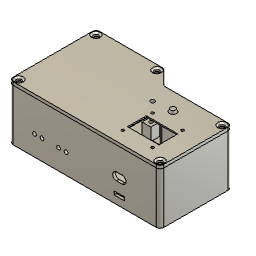
Blender_Box (Autodesk Fusion 360 design; units mm, degrees)
Autodesk Fusion 360 part; units mm, degrees
note: some values were not read from the file. Set by a fixed rule: which face or edge a step refers to.
sketch "Sketch1" plane through (0, 0, 0) normal (0, 1, 0) x (1, 0, 0)
  line L0 (0, 0) -> (120, 0)
  line L1 (0, 0) -> (0, 69)
  line L2 (0, 69) -> (54, 69)
  line L3 (54, 69) -> (66, 57)
  line L4 (66, 57) -> (120, 57)
  line L5 (120, 57) -> (120, 0)
  line L6 (54, 69) -> (54, 0) construction
  line L7 (66, 57) -> (66, 0) construction
  dimension "d1" = 120
  dimension "d2" = 69
  dimension "d3" = 54
  dimension "d5" = 57
  dimension "d28" = 54
  constraint coincident L0.start L1.start
  constraint horizontal L0
  constraint perpendicular L0 L1
  constraint perpendicular L1 L2
  constraint perpendicular L1 L4
  constraint perpendicular L0 L5
  constraint perpendicular L0 L6
  constraint coincident L0 L7.end
  constraint perpendicular L0 L7
  measures "d1" distance of L0.start L0.end
  measures "d2" distance of L0 L2
  measures "d3" distance of L1 L6
  measures "d5" distance of L0 L4
  measures "d28" distance of L5 L7
extrude "Extrude1" add sketch "Sketch1" along normal blind 41 makes body 1
shell "Shell1" thickness 2 removed faces 1 at (62, 41, -19) on bodies 1
sketch "Sketch2" plane through (0, 41, 0) normal (0, 1, 0) x (-1, 0, 0)
  line L0 (-2, -2) -> (-2, -67)
  line L1 (-2, -67) -> (-53.1716, -67)
  line L2 (-53.1716, -67) -> (-65.1716, -55)
  line L3 (-65.1716, -55) -> (-118, -55)
  line L4 (-118, -55) -> (-118, -2)
  line L5 (-118, -2) -> (-2, -2)
  line L6 (0, 0) -> (-120, 0)
  line L7 (-120, 0) -> (-120, -57)
  line L8 (-120, -57) -> (-66, -57)
  line L9 (-66, -57) -> (-54, -69)
  line L10 (-54, -69) -> (0, -69)
  line L11 (0, -69) -> (0, 0)
  circle A0 centre (-3.85, -3.85) radius 1.85
  circle A1 centre (-3.85, -65.15) radius 1.85
  circle A2 centre (-52.4053, -65.15) radius 1.85
  circle A3 centre (-116.15, -53.15) radius 1.85
  circle A4 centre (-116.15, -3.85) radius 1.85
  circle A5 centre (-3.85, -65.15) radius 3.85
  circle A6 centre (-52.4053, -65.15) radius 3.85
  circle A7 centre (-3.85, -3.85) radius 3.85
  circle A8 centre (-116.15, -53.15) radius 3.85
  circle A9 centre (-116.15, -3.85) radius 3.85
  dimension "d10" = 3.7
  constraint tangent L4 A4
  constraint tangent L5 A4
  constraint tangent L3 A3
  constraint tangent L4 A3
  constraint tangent L1 A2
  constraint tangent L2 A2
  constraint tangent L1 A1
  constraint tangent L0 A1
  constraint tangent L0 A0
  constraint tangent L5 A0
  constraint equal A0 A1
  constraint equal A0 A2
  constraint equal A2 A3
  constraint equal A3 A4
  constraint concentric A1 A5
  constraint concentric A2 A6
  constraint concentric A0 A7
  constraint concentric A3 A8
  constraint concentric A4 A9
  constraint tangent L7 A9
  constraint tangent L8 A8
  constraint tangent L9 A6
  constraint tangent L10 A5
  constraint tangent L11 A7
  measures "d10" diameter of A2
extrude "Extrude2" add sketch "Sketch2" against normal up to surface (39 mm away) contours L0 L5 A0 | L0 L5 A0 A7 | L0 L1 A1 A5 | L4 L5 A4 A9 | L0 L1 A1 | L4 L5 A4 | L1 L2 A2 A6 | L1 L2 A2 | L3 L4 A3 A8 | L3 L4 A3 bodies 1
fillet "Fillet1" radius 3 17 edges at (7.2264, 21.5, -67) (2, 21.5, -61.7736) (49.0289, 21.5, -67) (56.1009, 21.5, -64.0707) (65.1716, 21.5, -55) (112.7736, 21.5, -55) (118, 21.5, -49.7736) (0, 20.5, 0) (0, 20.5, -69) (54, 20.5, -69) (66, 20.5, -57) (120, 20.5, -57) (112.7736, 21.5, -2) (118, 21.5, -7.2264) (120, 20.5, 0) (7.2264, 21.5, -2) (2, 21.5, -7.2264) on bodies 1
sketch "Sketch4" plane through (0, 41, 0) normal (0, 1, 0) x (-1, 0, 0)
  arc A0 (-117, 0) -> (-120, -3) centre (-117, -3) ccw
  line L0 (-120, -3) -> (-120, -54)
  arc A1 (-120, -54) -> (-117, -57) centre (-117, -54) ccw
  line L1 (-117, -57) -> (-67.2426, -57)
  arc A2 (-65.1213, -57.8787) -> (-67.2426, -57) centre (-67.2426, -60) ccw
  line L2 (-65.1213, -57.8787) -> (-54.8787, -68.1213)
  arc A3 (-54.8787, -68.1213) -> (-52.7574, -69) centre (-52.7574, -66) ccw
  line L3 (-52.7574, -69) -> (-3, -69)
  arc A4 (-3, -69) -> (0, -66) centre (-3, -66) ccw
  line L4 (0, -66) -> (0, -3)
  arc A5 (0, -3) -> (-3, 0) centre (-3, -3) ccw
  line L5 (-3, 0) -> (-117, 0)
  circle A6 centre (-116.15, -3.85) radius 1.85
  circle A7 centre (-3.85, -65.15) radius 1.85
  circle A8 centre (-3.85, -3.85) radius 1.85
  circle A9 centre (-52.4053, -65.15) radius 1.85
  circle A10 centre (-116.15, -53.15) radius 1.85
  arc A11 (-64.2929, -55.8787) -> (-66.4142, -55) centre (-66.4142, -58) ccw
  line L6 (-66.4142, -55) -> (-109.3972, -55)
  arc A12 (-112.3546, -52.5036) -> (-109.3972, -55) centre (-109.3972, -52) ccw
  arc A13 (-112.3546, -52.5036) -> (-115.5036, -49.3546) centre (-116.15, -53.15) ccw
  arc A14 (-118, -46.3972) -> (-115.5036, -49.3546) centre (-115, -46.3972) ccw
  line L7 (-118, -46.3972) -> (-118, -10.6028)
  arc A15 (-115.5036, -7.6454) -> (-118, -10.6028) centre (-115, -10.6028) ccw
  arc A16 (-115.5036, -7.6454) -> (-112.3546, -4.4964) centre (-116.15, -3.85) ccw
  arc A17 (-109.3972, -2) -> (-112.3546, -4.4964) centre (-109.3972, -5) ccw
  line L8 (-109.3972, -2) -> (-10.6028, -2)
  arc A18 (-7.6454, -4.4964) -> (-4.4964, -7.6454) centre (-3.85, -3.85) ccw
  line L9 (-2, -10.6028) -> (-2, -58.3972)
  arc A19 (-4.4964, -61.3546) -> (-2, -58.3972) centre (-5, -58.3972) ccw
  arc A20 (-4.4964, -61.3546) -> (-7.6454, -64.5036) centre (-3.85, -65.15) ccw
  arc A21 (-10.6028, -67) -> (-7.6454, -64.5036) centre (-10.6028, -64) ccw
  line L10 (-10.6028, -67) -> (-45.6525, -67)
  arc A22 (-48.6099, -64.5036) -> (-45.6525, -67) centre (-45.6525, -64) ccw
  arc A23 (-48.6099, -64.5036) -> (-54.632, -62.0092) centre (-52.4053, -65.15) ccw
  arc A24 (-58.4884, -61.6832) -> (-54.632, -62.0092) centre (-56.367, -59.5619) ccw
  line L11 (-58.4884, -61.6832) -> (-64.2929, -55.8787)
  arc A25 (-7.6454, -4.4964) -> (-10.6028, -2) centre (-10.6028, -5) ccw
  arc A26 (-2, -10.6028) -> (-4.4964, -7.6454) centre (-5, -10.6028) ccw
extrude "Extrude1'" add sketch "Sketch4" along normal blind 2.5 separate body contours A0 L0 A1 L1 A2 L2 A3 L3 A4 L4 A5 L5 | A6 | A7 | A8 | A9 | A10 | A11 L6 A12 A13 A14 L7 A15 A16 A17 L8 A18 L9 A19 A20 A21 L10 A22 A23 A24 L11 A25 A26 makes body 2 in component "Lid"
sketch "Sketch1 (2)" plane through (0, 43.5, 0) normal (0, 1, 0) x (-1, 0, 0) in component "Lid"
  line L0 (-65.1213, -57.8787) -> (-54.8787, -68.1213)
  arc A0 (-54.8787, -68.1213) -> (-52.7574, -69) centre (-52.7574, -66) ccw
  line L1 (-52.7574, -69) -> (-3, -69)
  arc A1 (-3, -69) -> (0, -66) centre (-3, -66) ccw
  line L2 (0, -66) -> (0, -3)
  arc A2 (0, -3) -> (-3, 0) centre (-3, -3) ccw
  line L3 (-3, 0) -> (-117, 0)
  arc A3 (-117, 0) -> (-120, -3) centre (-117, -3) ccw
  line L4 (-120, -3) -> (-120, -54)
  arc A4 (-120, -54) -> (-117, -57) centre (-117, -54) ccw
  line L5 (-117, -57) -> (-67.2426, -57)
  arc A5 (-65.1213, -57.8787) -> (-67.2426, -57) centre (-67.2426, -60) ccw
  point P0 (-3.85, -3.85)
  point P1 (-3.85, -65.15)
  point P2 (-52.4053, -65.15)
  point P3 (-116.15, -3.85)
  point P4 (-116.15, -53.15)
hole "Hole1" at (116.15, 43.5, -53.15) at (116.15, 43.5, -3.85) at (52.4053, 43.5, -65.15) at (3.85, 43.5, -65.15) at (3.85, 43.5, -3.85) direction (0, -1, 0) diameter 4.5 depth 5 tip angle 118 countersink diameter 7 countersink angle 90 bodies 2 in component "Lid"
extrude "Extrude3" add sketch "Sketch4" against normal blind 2.5 draft -20 from surface at 2 contours A11 L6 A12 A13 A14 L7 A15 A16 A17 L8 A18 L9 A19 A20 A21 L10 A22 A23 A24 L11 A25 A26 bodies 2 in component "Lid"
sketch "Sketch2 (2)" plane through (0, 43.5, 0) normal (0, 1, 0) x (-1, 0, 0) in component "Lid"
  circle A0 centre (-3.85, -65.15) radius 3.5
  circle A1 centre (-116.15, -3.85) radius 3.5
  circle A2 centre (-116.15, -53.15) radius 3.5
  circle A3 centre (-52.4053, -65.15) radius 3.5
  circle A4 centre (-3.85, -3.85) radius 3.5
  line L0 (-65.1213, -57.8787) -> (-54.8787, -68.1213)
  arc A5 (-54.8787, -68.1213) -> (-52.7574, -69) centre (-52.7574, -66) ccw
  line L1 (-52.7574, -69) -> (-3, -69)
  arc A6 (-3, -69) -> (0, -66) centre (-3, -66) ccw
  line L2 (0, -66) -> (0, -3)
  arc A7 (0, -3) -> (-3, 0) centre (-3, -3) ccw
  line L3 (-3, 0) -> (-117, 0)
  arc A8 (-117, 0) -> (-120, -3) centre (-117, -3) ccw
  line L4 (-120, -3) -> (-120, -54)
  arc A9 (-120, -54) -> (-117, -57) centre (-117, -54) ccw
  line L5 (-117, -57) -> (-67.2426, -57)
  arc A10 (-65.1213, -57.8787) -> (-67.2426, -57) centre (-67.2426, -60) ccw
  line L6 (-104.6213, -29.5) -> (-79.6213, -29.5)
  line L7 (-79.6213, -29.5) -> (-79.6213, -14.5)
  line L8 (-79.6213, -14.5) -> (-104.6213, -14.5)
  line L9 (-104.6213, -14.5) -> (-104.6213, -29.5)
  line L10 (-104.6213, -29.5) -> (-79.6213, -14.5) construction
  line L11 (-79.6213, -29.5) -> (-104.6213, -14.5) construction
  line L12 (-92.1213, -22) -> (-120, -22) construction
  line L13 (-92.1213, -22) -> (-92.1213, -57) construction
  circle A11 centre (-80.2213, -33.9) radius 1.1
  circle A12 centre (-104.0213, -33.9) radius 1.1
  circle A13 centre (-104.0213, -10.1) radius 1.1
  circle A14 centre (-80.2213, -10.1) radius 1.1
  line L14 (-80.2213, -33.9) -> (-104.0213, -10.1) construction
  circle A15 centre (-72.1213, -42) radius 1.65
  point P0 (-92.1213, -22)
  point P1 (-92.1213, -22)
  dimension "d29" = 15
  dimension "d30" = 25
  dimension "d31" = 23.8
  dimension "d32" = 23.8
  dimension "d33" = 2.2
  dimension "d39" = 3.3
  dimension "d40" = 20
  dimension "d67" = 35
  dimension "d68" = 20
  constraint horizontal L6
  constraint perpendicular L6 L7
  constraint parallel L6 L8
  constraint parallel L7 L9
  constraint coincident L10 P1
  constraint coincident L11 P1
  constraint coincident P1 P0
  constraint horizontal L12
  constraint midpoint L5 L13.end
  constraint vertical L13
  constraint horizontal A11.centre A12.centre
  constraint vertical A11.centre A14.centre
  constraint vertical A12.centre A13.centre
  constraint horizontal A13.centre A14.centre
  constraint coincident A11.centre L14.start
  constraint coincident A13.centre L14.end
  constraint midpoint L14 P1
  constraint equal A11 A12
  constraint equal A11 A14
  constraint equal A13 A14
  measures "d29" distance of L6.end L7.end
  measures "d30" distance of L7 L9
  measures "d31" distance of A11.centre A12.centre
  measures "d32" distance of A11.centre A14.centre
  measures "d33" diameter of A11
  measures "d39" diameter of A15
  measures "d40" horizontal distance of P1 A15.centre
  measures "d67" distance of L12 L13.end
  measures "d68" distance of L12 A15.centre
extrude "Extrude4" cut sketch "Sketch2 (2)" against normal through all contours L6 L7 L8 L9 | A11 | A12 | A13 | A14 | A15 bodies 2 in component "Lid"
sketch "Sketch3" plane through (0, 40.5, 0) normal (0, -1, 0) x (1, 0, 0) in component "Lid"
  circle A0 centre (104.0213, -33.9) radius 1.1
  circle A1 centre (80.2213, -33.9) radius 1.1
  circle A2 centre (80.2213, -10.1) radius 1.1
  line L0 (79.6213, -14.5) -> (104.6213, -14.5)
  line L1 (104.6213, -14.5) -> (104.6213, -29.5)
  line L2 (104.6213, -29.5) -> (79.6213, -29.5)
  line L3 (79.6213, -29.5) -> (79.6213, -14.5)
  circle A3 centre (104.0213, -10.1) radius 1.1
  arc A4 (2.9099, -58.3972) -> (4.6491, -60.4576) centre (5, -58.3972) ccw
  arc A5 (8.5424, -64.3509) -> (4.6491, -60.4576) centre (3.85, -65.15) ccw
  arc A6 (8.5424, -64.3509) -> (10.6028, -66.0901) centre (10.6028, -64) ccw
  line L4 (10.6028, -66.0901) -> (45.6525, -66.0901)
  arc A7 (45.6525, -66.0901) -> (47.7129, -64.3509) centre (45.6525, -64) ccw
  arc A8 (55.1582, -61.2669) -> (47.7129, -64.3509) centre (52.4053, -65.15) ccw
  arc A9 (55.1582, -61.2669) -> (57.8449, -61.0398) centre (56.367, -59.5619) ccw
  line L5 (57.8449, -61.0398) -> (63.6495, -55.2353)
  arc A10 (66.4142, -54.0901) -> (63.6495, -55.2353) centre (66.4142, -58) ccw
  line L6 (66.4142, -54.0901) -> (109.3972, -54.0901)
  arc A11 (109.3972, -54.0901) -> (111.4576, -52.3509) centre (109.3972, -52) ccw
  arc A12 (115.3509, -48.4576) -> (111.4576, -52.3509) centre (116.15, -53.15) ccw
  arc A13 (115.3509, -48.4576) -> (117.0901, -46.3972) centre (115, -46.3972) ccw
  line L7 (117.0901, -46.3972) -> (117.0901, -10.6028)
  arc A14 (117.0901, -10.6028) -> (115.3509, -8.5424) centre (115, -10.6028) ccw
  arc A15 (111.4576, -4.6491) -> (115.3509, -8.5424) centre (116.15, -3.85) ccw
  arc A16 (111.4576, -4.6491) -> (109.3972, -2.9099) centre (109.3972, -5) ccw
  line L8 (109.3972, -2.9099) -> (10.6028, -2.9099)
  arc A17 (10.6028, -2.9099) -> (8.5424, -4.6491) centre (10.6028, -5) ccw
  arc A18 (4.6491, -8.5424) -> (8.5424, -4.6491) centre (3.85, -3.85) ccw
  arc A19 (4.6491, -8.5424) -> (2.9099, -10.6028) centre (5, -10.6028) ccw
  line L9 (2.9099, -10.6028) -> (2.9099, -58.3972)
  line L10 (106.1213, -11.2) -> (78.1213, -11.2)
  line L11 (78.1213, -11.2) -> (78.1213, -32.8)
  line L12 (78.1213, -32.8) -> (106.1213, -32.8)
  line L13 (106.1213, -32.8) -> (106.1213, -11.2)
  line L14 (106.1213, -11.2) -> (78.1213, -32.8) construction
  line L15 (78.1213, -11.2) -> (106.1213, -32.8) construction
  line L16 (81.3213, -8) -> (102.9213, -8)
  line L17 (102.9213, -8) -> (102.9213, -36)
  line L18 (102.9213, -36) -> (81.3213, -36)
  line L19 (81.3213, -36) -> (81.3213, -8)
  line L20 (81.3213, -8) -> (102.9213, -36) construction
  line L21 (102.9213, -8) -> (81.3213, -36) construction
  line L22 (79.1213, -11.2) -> (79.1213, -9) construction
  line L23 (79.1213, -9) -> (81.3213, -9) construction
  line L24 (78.1213, -11.2) -> (78.1213, -8)
  line L25 (78.1213, -8) -> (81.3213, -8)
  line L26 (102.9213, -8) -> (106.1213, -8)
  line L27 (106.1213, -8) -> (106.1213, -11.2)
  line L28 (106.1213, -32.8) -> (106.1213, -36)
  line L29 (106.1213, -36) -> (102.9213, -36)
  line L30 (81.3213, -36) -> (78.1213, -36)
  line L31 (78.1213, -36) -> (78.1213, -32.8)
  circle A20 centre (72.1213, -42) radius 1.65
  point P0 (92.1213, -22)
  point P1 (92.1213, -22)
  point P2 (92.1213, -22)
  dimension "d35" = 1
  dimension "d36" = 1
  constraint horizontal L10
  constraint perpendicular L10 L11
  constraint parallel L10 L12
  constraint parallel L11 L13
  constraint coincident L14 P2
  constraint coincident L15 P2
  constraint coincident P2 P1
  constraint horizontal L16
  constraint perpendicular L16 L17
  constraint parallel L16 L18
  constraint parallel L17 L19
  constraint coincident L20 P2
  constraint coincident L21 P2
  constraint tangent A2 L19
  constraint coincident L10 L22.start
  constraint parallel L10 L23
  constraint coincident L19 L23.end
  constraint tangent A2 L23
  constraint tangent A2 L22
  constraint vertical L22
  constraint tangent A2 L10
  constraint perpendicular L16 L24
  constraint perpendicular L19 L25
  constraint perpendicular L13 L26
  constraint perpendicular L10 L27
  constraint perpendicular L18 L28
  constraint perpendicular L17 L29
  constraint perpendicular L11 L30
  constraint perpendicular L12 L31
  measures "d35" distance of L16 L23
  measures "d36" distance of L11 L22.start
extrude "Extrude5" cut sketch "Sketch3" against normal blind 2 contours A0 L12 L17 | L0 L1 L2 L10 L12 L13 L17 | L12 L17 L18 L19 | L2 L12 L17 L19 | A1 L12 L19 | L0 L2 L3 L10 L11 L12 L19 | L0 L10 L17 L19 | A3 L10 L17 | L10 L16 L17 L19 | A2 L10 L19 bodies 2 in component "Lid"
sketch "Sketch5" plane through (0, 2, 0) normal (0, 1, 0) x (-1, 0, 0)
  arc A0 (-2, -10.6028) -> (-4.4964, -7.6454) centre (-5, -10.6028) ccw
  arc A1 (-7.6454, -4.4964) -> (-4.4964, -7.6454) centre (-3.85, -3.85) ccw
  arc A2 (-7.6454, -4.4964) -> (-10.6028, -2) centre (-10.6028, -5) ccw
  line L0 (-10.6028, -2) -> (-109.3972, -2)
  arc A3 (-109.3972, -2) -> (-112.3546, -4.4964) centre (-109.3972, -5) ccw
  arc A4 (-115.5036, -7.6454) -> (-112.3546, -4.4964) centre (-116.15, -3.85) ccw
  arc A5 (-115.5036, -7.6454) -> (-118, -10.6028) centre (-115, -10.6028) ccw
  line L1 (-118, -10.6028) -> (-118, -46.3972)
  arc A6 (-118, -46.3972) -> (-115.5036, -49.3546) centre (-115, -46.3972) ccw
  arc A7 (-112.3546, -52.5036) -> (-115.5036, -49.3546) centre (-116.15, -53.15) ccw
  arc A8 (-112.3546, -52.5036) -> (-109.3972, -55) centre (-109.3972, -52) ccw
  line L2 (-109.3972, -55) -> (-66.4142, -55)
  arc A9 (-64.2929, -55.8787) -> (-66.4142, -55) centre (-66.4142, -58) ccw
  line L3 (-64.2929, -55.8787) -> (-58.4884, -61.6832)
  arc A10 (-58.4884, -61.6832) -> (-54.632, -62.0092) centre (-56.367, -59.5619) ccw
  arc A11 (-48.6099, -64.5036) -> (-54.632, -62.0092) centre (-52.4053, -65.15) ccw
  arc A12 (-48.6099, -64.5036) -> (-45.6525, -67) centre (-45.6525, -64) ccw
  line L4 (-45.6525, -67) -> (-10.6028, -67)
  arc A13 (-10.6028, -67) -> (-7.6454, -64.5036) centre (-10.6028, -64) ccw
  arc A14 (-4.4964, -61.3546) -> (-7.6454, -64.5036) centre (-3.85, -65.15) ccw
  arc A15 (-4.4964, -61.3546) -> (-2, -58.3972) centre (-5, -58.3972) ccw
  line L5 (-2, -58.3972) -> (-2, -10.6028)
  line L6 (-65.3, -49) -> (-112.3, -49) construction
  line L7 (-112.3, -49) -> (-112.3, -2) construction
  line L8 (-112.3, -2) -> (-65.3, -2) construction
  line L9 (-65.3, -2) -> (-65.3, -49) construction
  line L10 (-65.3, -2) -> (-73.3, -2)
  line L11 (-73.3, -2) -> (-73.3, -8.9)
  line L12 (-73.3, -8.9) -> (-65.3, -8.9)
  line L13 (-65.3, -8.9) -> (-65.3, -2)
  line L14 (-112.3, -2) -> (-104.3, -2)
  line L15 (-104.3, -2) -> (-104.3, -8.9)
  line L16 (-104.3, -8.9) -> (-112.3, -8.9)
  line L17 (-112.3, -8.9) -> (-112.3, -2)
  line L18 (-112.3, -49) -> (-65.3, -49)
  line L19 (-65.3, -49) -> (-65.3, -44)
  line L20 (-65.3, -44) -> (-112.3, -44)
  line L21 (-112.3, -44) -> (-112.3, -49)
  dimension "d42" = 47
  dimension "d43" = 47
  dimension "d44" = 8
  dimension "d45" = 6.9
  dimension "d56" = 5
  constraint horizontal L6
  constraint vertical L7
  constraint horizontal L8
  constraint vertical L9
  constraint coincident L7.end L8.start
  constraint coincident L0 L8.end
  constraint tangent A4 L7
  constraint horizontal L10
  constraint vertical L11
  constraint horizontal L12
  constraint vertical L13
  constraint horizontal L14
  constraint vertical L15
  constraint horizontal L16
  constraint vertical L17
  constraint equal L12 L16
  constraint equal L11 L15
  constraint horizontal L18
  constraint vertical L19
  constraint horizontal L20
  constraint vertical L21
  constraint coincident L9 L19.end
  measures "d42" distance of L6.start L6.end
  measures "d43" distance of L6 L8
  measures "d44" distance of L11.end L12.end
  measures "d45" distance of L10.end L11.end
  measures "d56" distance of L6 L20
extrude "Extrude3'" add sketch "Sketch5" along normal blind 10 contours L0 L10 L11 L12 L13 | L0 A3 L14 L15 L16 L17 | L18 L19 L20 L21 bodies 1
sketch "Sketch6" plane through (0, 41, 0) normal (0, 1, 0) x (-1, 0, 0)
  arc A0 (-117, 0) -> (-120, -3) centre (-117, -3) ccw
  line L0 (-120, -3) -> (-120, -54)
  arc A1 (-120, -54) -> (-117, -57) centre (-117, -54) ccw
  line L1 (-117, -57) -> (-67.2426, -57)
  arc A2 (-65.1213, -57.8787) -> (-67.2426, -57) centre (-67.2426, -60) ccw
  line L2 (-65.1213, -57.8787) -> (-54.8787, -68.1213)
  arc A3 (-54.8787, -68.1213) -> (-52.7574, -69) centre (-52.7574, -66) ccw
  line L3 (-52.7574, -69) -> (-3, -69)
  arc A4 (-3, -69) -> (0, -66) centre (-3, -66) ccw
  line L4 (0, -66) -> (0, -3)
  arc A5 (0, -3) -> (-3, 0) centre (-3, -3) ccw
  line L5 (-3, 0) -> (-117, 0)
  circle A6 centre (-116.15, -3.85) radius 1.85
  circle A7 centre (-3.85, -65.15) radius 1.85
  circle A8 centre (-3.85, -3.85) radius 1.85
  circle A9 centre (-52.4053, -65.15) radius 1.85
  circle A10 centre (-116.15, -53.15) radius 1.85
  arc A11 (-64.2929, -55.8787) -> (-66.4142, -55) centre (-66.4142, -58) ccw
  line L6 (-66.4142, -55) -> (-109.3972, -55)
  arc A12 (-112.3546, -52.5036) -> (-109.3972, -55) centre (-109.3972, -52) ccw
  arc A13 (-112.3546, -52.5036) -> (-115.5036, -49.3546) centre (-116.15, -53.15) ccw
  arc A14 (-118, -46.3972) -> (-115.5036, -49.3546) centre (-115, -46.3972) ccw
  line L7 (-118, -46.3972) -> (-118, -10.6028)
  arc A15 (-115.5036, -7.6454) -> (-118, -10.6028) centre (-115, -10.6028) ccw
  arc A16 (-115.5036, -7.6454) -> (-112.3546, -4.4964) centre (-116.15, -3.85) ccw
  arc A17 (-109.3972, -2) -> (-112.3546, -4.4964) centre (-109.3972, -5) ccw
  line L8 (-109.3972, -2) -> (-10.6028, -2)
  arc A18 (-7.6454, -4.4964) -> (-10.6028, -2) centre (-10.6028, -5) ccw
  arc A19 (-7.6454, -4.4964) -> (-4.4964, -7.6454) centre (-3.85, -3.85) ccw
  arc A20 (-2, -10.6028) -> (-4.4964, -7.6454) centre (-5, -10.6028) ccw
  line L9 (-2, -10.6028) -> (-2, -58.3972)
  arc A21 (-4.4964, -61.3546) -> (-2, -58.3972) centre (-5, -58.3972) ccw
  arc A22 (-4.4964, -61.3546) -> (-7.6454, -64.5036) centre (-3.85, -65.15) ccw
  arc A23 (-10.6028, -67) -> (-7.6454, -64.5036) centre (-10.6028, -64) ccw
  line L10 (-10.6028, -67) -> (-45.6525, -67)
  arc A24 (-48.6099, -64.5036) -> (-45.6525, -67) centre (-45.6525, -64) ccw
  arc A25 (-48.6099, -64.5036) -> (-54.632, -62.0092) centre (-52.4053, -65.15) ccw
  arc A26 (-58.4884, -61.6832) -> (-54.632, -62.0092) centre (-56.367, -59.5619) ccw
  line L11 (-58.4884, -61.6832) -> (-64.2929, -55.8787)
  line L12 (-104.3, -8.9) -> (-112.3, -8.9)
  line L13 (-112.3, -8.9) -> (-112.3, -2)
  line L14 (-112.3, -2) -> (-104.3, -2)
  line L15 (-104.3, -2) -> (-104.3, -8.9)
  line L16 (-112.3, -4.2424) -> (-112.3, -8.9)
  point P0 (-104.3, -8.9)
  point P1 (-109.3972, -2)
  constraint horizontal L12
  constraint vertical L13
  constraint horizontal L14
  constraint vertical L15
  constraint coincident P0 L12.start
  constraint coincident L14 P1
  constraint coincident L13 L16.start
extrude "Extrude4'" cut sketch "Sketch6" against normal up to surface (29 mm away) contours A17 L13 L14 bodies 1
sketch "Sketch7" plane through (0, 12, 0) normal (0, 1, 0) x (-1, 0, 0)
  line L0 (-112.3, -4.2424) -> (-112.3, -8.9)
  line L1 (-112.3, -8.9) -> (-104.3, -8.9)
  line L2 (-104.3, -8.9) -> (-104.3, -2)
  line L3 (-104.3, -2) -> (-112.3, -2)
  line L4 (-112.3, -2) -> (-112.3, -4.2424)
  circle A0 centre (-108, -5) radius 1.4
  circle A1 centre (-70, -5) radius 1.4
  line L5 (-112.3, -2) -> (-10.6028, -2)
  dimension "d50" = 38
  dimension "d51" = 2.8
  dimension "d52" = 4.3
  dimension "d53" = 3
  constraint horizontal A0.centre A1.centre
  constraint equal A0 A1
  measures "d50" distance of A0.centre A1.centre
  measures "d51" diameter of A0
  measures "d52" distance of L0 A0.centre
  measures "d53" distance of A0.centre L5
extrude "Extrude5'" cut sketch "Sketch7" against normal blind 10 contours A0 | A1 bodies 1
extrude "Extrude6" cut 1 faces at (80.9667, 12, -47.3333) along direction (0, -1, 0) blind 2.7 on bodies 1 bodies 1
sketch "Sketch8" plane through (0, 0, -2) normal (0, 0, -1) x (-1, 0, 0)
  line L0 (-65.3, 12) -> (-65.3, 2)
  line L1 (-65.3, 2) -> (-10.6028, 2)
  line L2 (-10.6028, 2) -> (-10.6028, 41)
  line L3 (-10.6028, 41) -> (-112.3, 41)
  line L4 (-112.3, 41) -> (-112.3, 12)
  line L5 (-112.3, 12) -> (-104.3, 12)
  line L6 (-104.3, 12) -> (-104.3, 2)
  line L7 (-104.3, 2) -> (-73.3, 2)
  line L8 (-73.3, 2) -> (-73.3, 12)
  line L9 (-73.3, 12) -> (-65.3, 12)
  line L10 (-89.85, 16.3) -> (-85.35, 16.3)
  arc A0 (-85.35, 16.3) -> (-85.35, 22.4) centre (-85.35, 19.35) ccw
  line L11 (-85.35, 22.4) -> (-89.85, 22.4)
  arc A1 (-89.85, 22.4) -> (-89.85, 16.3) centre (-89.85, 19.35) ccw
  line L12 (-92.9, 19.35) -> (-82.3, 19.35) construction
  line L13 (-82.3, 19.35) -> (-82.3, 12) construction
  line L14 (-112.3, 12) -> (-104.3, 12) construction
  line L15 (-91.6, 8.35) -> (-83.6, 8.35)
  line L16 (-83.6, 8.35) -> (-83.6, 5.65)
  line L17 (-83.6, 5.65) -> (-91.6, 5.65)
  line L18 (-91.6, 5.65) -> (-91.6, 8.35)
  line L19 (-91.6, 8.35) -> (-83.6, 5.65) construction
  line L20 (-87.6, 19.35) -> (-87.6, 7) construction
  point P0 (-104.3, 12)
  point P1 (-112.3, 12)
  dimension "d59" = 4.3
  dimension "d60" = 10.6
  dimension "d61" = 6.1
  dimension "d62" = 30
  dimension "d63" = 2.7
  dimension "d64" = 8
  dimension "d65" = 11
  constraint tangent L10 A0
  constraint tangent A0 L11
  constraint parallel L10 L11
  constraint tangent L11 A1
  constraint tangent L10 A1
  constraint midpoint A1 L12.start
  constraint midpoint A0 L12.end
  constraint tangent A0 L13
  constraint perpendicular L12 L13
  constraint coincident P1 L4.end
  constraint coincident P0 L5.end
  constraint coincident L13.end L14
  constraint horizontal L15
  constraint vertical L16
  constraint horizontal L17
  constraint vertical L18
  constraint midpoint L12 L20.start
  constraint midpoint L19 L20.end
  constraint vertical L20
  measures "d59" distance of L9 L10
  measures "d60" distance of L12.start L12.end
  measures "d61" distance of L10 L11
  measures "d62" distance of L13 P1
  measures "d63" distance of L15 L17
  measures "d64" distance of L15.start L15.end
  measures "d65" distance of L12 L15
extrude "Extrude7" cut sketch "Sketch8" against normal through all contours L10 A0 L11 A1 | L15 L16 L17 L18 bodies 1
sketch "Sketch4 (2)" plane through (0, 43.5, 0) normal (0, 1, 0) x (-1, 0, 0) in component "Lid"
  circle A0 centre (-80.2213, -10.1) radius 1.1
  line L0 (-104.6213, -14.5) -> (-79.6213, -14.5)
  line L1 (-79.6213, -14.5) -> (-79.6213, -29.5)
  line L2 (-79.6213, -29.5) -> (-104.6213, -29.5)
  line L3 (-104.6213, -29.5) -> (-104.6213, -14.5)
  circle A1 centre (-104.0213, -10.1) radius 1.1
  circle A2 centre (-104.0213, -33.9) radius 1.1
  circle A3 centre (-80.2213, -33.9) radius 1.1
  circle A4 centre (-72.1213, -42) radius 1.65
  circle A5 centre (-3.85, -65.15) radius 3.5
  circle A6 centre (-116.15, -3.85) radius 3.5
  circle A7 centre (-116.15, -53.15) radius 3.5
  circle A8 centre (-52.4053, -65.15) radius 3.5
  circle A9 centre (-3.85, -3.85) radius 3.5
  line L4 (-65.1213, -57.8787) -> (-54.8787, -68.1213)
  arc A10 (-54.8787, -68.1213) -> (-52.7574, -69) centre (-52.7574, -66) ccw
  line L5 (-52.7574, -69) -> (-3, -69)
  arc A11 (-3, -69) -> (0, -66) centre (-3, -66) ccw
  line L6 (0, -66) -> (0, -3)
  arc A12 (0, -3) -> (-3, 0) centre (-3, -3) ccw
  line L7 (-3, 0) -> (-117, 0)
  arc A13 (-117, 0) -> (-120, -3) centre (-117, -3) ccw
  line L8 (-120, -3) -> (-120, -54)
  arc A14 (-120, -54) -> (-117, -57) centre (-117, -54) ccw
  line L9 (-117, -57) -> (-67.2426, -57)
  arc A15 (-65.1213, -57.8787) -> (-67.2426, -57) centre (-67.2426, -60) ccw
  line L10 (-112.3, -49) -> (-112.3, -2)
  line L11 (-112.3, -2) -> (-65.3, -2)
  circle A16 centre (-87.3, -43) radius 2
  circle A17 centre (-87.3, -43) radius 2.8
  line L12 (-86.3, -43) -> (-88.3, -43)
  line L13 (-88.3, -43) -> (-88.3, -40.2)
  line L14 (-88.3, -40.2) -> (-86.3, -40.2)
  line L15 (-86.3, -40.2) -> (-86.3, -43)
  point P0 (-87.3, -43)
  point P1 (-87.3, -43)
  dimension "d69" = 25
  dimension "d70" = 41
  dimension "d71" = 4
  dimension "d72" = 0.8
  dimension "d73" = 2
  constraint coincident P1 P0
  constraint concentric A16 A17
  constraint horizontal L12
  constraint vertical L13
  constraint horizontal L14
  constraint vertical L15
  constraint midpoint L12 P1
  constraint tangent A17 L14
  measures "d69" distance of P1 L10
  measures "d70" distance of P1 L11
  measures "d71" diameter of A16
  measures "d72" distance of A16 A17
  measures "d73" distance of L13 L15
extrude "Extrude6'" cut sketch "Sketch4 (2)" against normal through all contours A16 L12 L13 L15 | A16 A17 L13 L15 | A16 L12 L13 L15 | A16 A17 L13 L15 bodies 2 in component "Lid"
sketch "Sketch9" plane through (60, 2, -34.5) normal (0, 1, 0) x (-1, 0, 0)
  line L0 (52.3, 32.5) -> (2.3, 32.5)
  line L1 (2.3, 32.5) -> (2.3, -27.5)
  line L2 (2.3, -27.5) -> (52.3, -27.5)
  line L3 (52.3, -27.5) -> (52.3, 32.5)
  line L4 (49.3972, 32.5) -> (-49.3972, 32.5)
  arc A0 (52.3546, 30.0036) -> (55.5036, 26.8546) centre (56.15, 30.65) ccw
  dimension "d77" = 50
  dimension "d78" = 60
  constraint horizontal L0
  constraint vertical L1
  constraint horizontal L2
  constraint vertical L3
  constraint coincident L0.start L4
  constraint tangent L3 A0
  measures "d77" distance of L0.start L0.end
  measures "d78" distance of L0.start L2.end
extrude "Extrude8" cut sketch "Sketch9" along normal through all bodies 1
sketch "Sketch10" plane through (60, 2, -34.5) normal (0, 1, 0) x (-1, 0, 0)
  line L0 (52.3, -27.5) -> (45.3, -27.5)
  line L1 (45.3, -27.5) -> (45.3, -20.5)
  line L2 (45.3, -20.5) -> (52.3, -20.5)
  line L3 (52.3, -20.5) -> (52.3, -27.5)
  line L4 (9.3, -27.5) -> (2.3, -27.5)
  line L5 (2.3, -27.5) -> (2.3, -20.5)
  line L6 (2.3, -20.5) -> (9.3, -20.5)
  line L7 (9.3, -20.5) -> (9.3, -27.5)
  line L8 (52.3, 25.5) -> (45.3, 25.5)
  line L9 (45.3, 25.5) -> (45.3, 32.5)
  line L10 (45.3, 32.5) -> (52.3, 32.5)
  line L11 (52.3, 32.5) -> (52.3, 25.5)
  line L12 (9.3, 25.5) -> (2.3, 25.5)
  line L13 (2.3, 25.5) -> (2.3, 32.5)
  line L14 (2.3, 32.5) -> (9.3, 32.5)
  line L15 (9.3, 32.5) -> (9.3, 25.5)
  line L16 (52.3, -27.5) -> (52.3, 32.5)
  line L17 (2.3, -27.5) -> (52.3, -27.5)
  circle A0 centre (48.8, -24.05) radius 1.35
  circle A1 centre (5.8, -24.05) radius 1.35
  circle A2 centre (48.8, 29.05) radius 1.35
  circle A3 centre (5.8, 29.05) radius 1.35
  line L18 (48.8, -24.05) -> (5.8, -24.05) construction
  line L19 (27.3, -24.05) -> (27.3, -27.5) construction
  line L20 (48.8, -24.05) -> (48.8, 29.05) construction
  line L21 (48.8, 2.5) -> (52.3, 2.5) construction
  point P0 (52.3, -27.5)
  point P1 (2.3, -27.5)
  point P2 (2.3, 32.5)
  point P3 (52.3, 32.5)
  dimension "d80" = 7
  dimension "d81" = 7
  dimension "d82" = 43
  dimension "d83" = 2.7
  dimension "d84" = 3.45
  constraint horizontal L0
  constraint vertical L1
  constraint horizontal L2
  constraint vertical L3
  constraint horizontal L4
  constraint vertical L5
  constraint horizontal L6
  constraint vertical L7
  constraint horizontal L8
  constraint vertical L9
  constraint horizontal L10
  constraint vertical L11
  constraint horizontal L12
  constraint vertical L13
  constraint horizontal L14
  constraint vertical L15
  constraint coincident P0 L0.start
  constraint coincident P1 L4.end
  constraint coincident P2 L13.end
  constraint coincident P3 L10.end
  constraint equal L1 L7
  constraint equal L7 L9
  constraint equal L9 L15
  constraint equal L2 L6
  constraint equal L6 L12
  constraint equal L8 L12
  constraint horizontal A0.centre A1.centre
  constraint vertical A0.centre A2.centre
  constraint vertical A1.centre A3.centre
  constraint horizontal A2.centre A3.centre
  constraint equal A0 A1
  constraint equal A1 A2
  constraint equal A2 A3
  constraint coincident A0.centre L18.start
  constraint coincident A1.centre L18.end
  constraint midpoint L18 L19.start
  constraint midpoint L17 L19.end
  constraint vertical L19
  constraint coincident A2.centre L20.end
  constraint midpoint L20 L21.start
  constraint midpoint L16 L21.end
  constraint horizontal L21
  measures "d80" distance of L1 L16
  measures "d81" distance of L2 L17
  measures "d82" distance of A0.centre A1.centre
  measures "d83" diameter of A0
  measures "d84" distance of L17 L18
extrude "Extrude9" add sketch "Sketch10" along normal blind 10 bodies 1
sketch "Sketch11" plane through (0, 0, 0) normal (0, 0, 1) x (1, 0, 0)
  line L0 (91.6, 8.35) -> (91.6, 5.65)
  line L1 (91.6, 5.65) -> (83.6, 5.65)
  line L2 (83.6, 5.65) -> (83.6, 8.35)
  line L3 (83.6, 8.35) -> (91.6, 8.35)
  line L4 (85.35, 22.4) -> (89.85, 22.4)
  arc A0 (89.85, 16.3) -> (89.85, 22.4) centre (89.85, 19.35) ccw
  line L5 (89.85, 16.3) -> (85.35, 16.3)
  arc A1 (85.35, 22.4) -> (85.35, 16.3) centre (85.35, 19.35) ccw
  line L6 (117, 0) -> (117, 41)
  line L7 (117, 41) -> (3, 41)
  line L8 (3, 41) -> (3, 0)
  line L9 (3, 0) -> (117, 0)
  line L10 (7.7, 12) -> (14.7, 12)
  line L11 (50.7, 12) -> (57.7, 12)
  circle A2 centre (20.125, 16) radius 1.5
  circle A3 centre (26.125, 16) radius 1.5
  circle A4 centre (39.275, 16) radius 1.5
  circle A5 centre (45.275, 16) radius 1.5
  line L12 (20.125, 16) -> (26.125, 16) construction
  line L13 (26.125, 16) -> (39.275, 16) construction
  line L14 (39.275, 16) -> (45.275, 16) construction
  line L15 (14.7, 12) -> (50.7, 12) construction
  line L16 (32.7, 16) -> (32.7, 12) construction
  point P0 (23.125, 16)
  point P1 (42.275, 16)
  dimension "d87" = 4
  dimension "d88" = 3
  dimension "d89" = 6
  dimension "d90" = 19.15
  constraint coincident A2.centre L12.start
  constraint coincident A3.centre L12.end
  constraint horizontal L12
  constraint coincident A4.centre L13.end
  constraint parallel L12 L13
  constraint coincident A5.centre L14.end
  constraint parallel L13 L14
  constraint equal L12 L14
  constraint equal A2 A3
  constraint equal A4 A5
  constraint equal A3 A4
  constraint coincident L10.end L15.start
  constraint coincident L11.start L15.end
  constraint midpoint L13 L16.start
  constraint midpoint L15 L16.end
  constraint vertical L16
  constraint midpoint L12 P0
  constraint midpoint L14 P1
  measures "d87" distance of L10 A2.centre
  measures "d88" diameter of A2
  measures "d89" distance of A2.centre A3.centre
  measures "d90" distance of P0 P1
extrude "Extrude10" cut sketch "Sketch11" against normal up to surface (55 mm away) contours A2 | A3 | A4 | A5 bodies 1
extrude "Extrude11" add sketch "Sketch4 (2)" along normal blind 2 and the other way blind 30 separate body contours A16 L12 L13 L15 | A16 L12 L13 L15 makes body 3
copy_body "Body->Comp1" bodies 3 removing the originals makes body 4 in component "Button_Post"
component "Lid" placed x (1, 0, 0) y (0, 1, 0) z (0, 0, 1) at (0, 0, 0)
component "Button_Post" placed x (1, 0, 0) y (0, 1, 0) z (0, 0, 1) at (0, 0, 0)
equation "d2 = 63 mm + ( 2 * 3 ) * 1 mm"
equation "d3 = 51 mm + ( 1 * 3 ) * 1 mm"
equation "d5 = 51 mm + ( 3 * 2 ) * 1 mm"
equation "d7 = 35 mm + ( 2 * 3 ) * 1 mm"
equation "d28 = 51 mm + ( 1 * 3 ) * 1 mm"
equation "d36 = d35"
equation "d72 = d71 * 0.2"
equation "d73 = d71 / 2"
